Autodesk Inventor part; units mm, degrees
(part 3 of 3)
ref_plane "to_Bolt_1_6_YZ" through (-291.404, 0, -380) normal (1, 0, 0) x (0, 0, -1)
ref_plane "to_Bolt_1_6_ZX" through (-291.404, 0, -380) normal (0, 0, -1) x (0, 1, 0)
ref_plane "to_Bolt_1_60_XY" through (-198.5673, 0, -380) normal (0, 1, 0) x (1, 0, 0)
ref_plane "to_Bolt_1_60_YZ" through (-198.5673, 0, -380) normal (1, 0, 0) x (0, 0, -1)
ref_plane "to_Bolt_1_60_ZX" through (-198.5673, 0, -380) normal (0, 0, -1) x (0, 1, 0)
ref_plane "to_Bolt_1_61_XY" through (-196.8481, 0, -380) normal (0, 1, 0) x (1, 0, 0)
ref_plane "to_Bolt_1_61_YZ" through (-196.8481, 0, -380) normal (1, 0, 0) x (0, 0, -1)
ref_plane "to_Bolt_1_61_ZX" through (-196.8481, 0, -380) normal (0, 0, -1) x (0, 1, 0)
ref_plane "to_Bolt_1_62_XY" through (-195.1289, 0, -380) normal (0, 1, 0) x (1, 0, 0)
ref_plane "to_Bolt_1_62_YZ" through (-195.1289, 0, -380) normal (1, 0, 0) x (0, 0, -1)
ref_plane "to_Bolt_1_62_ZX" through (-195.1289, 0, -380) normal (0, 0, -1) x (0, 1, 0)
ref_plane "to_Bolt_1_63_XY" through (-193.4097, 0, -380) normal (0, 1, 0) x (1, 0, 0)
ref_plane "to_Bolt_1_63_YZ" through (-193.4097, 0, -380) normal (1, 0, 0) x (0, 0, -1)
ref_plane "to_Bolt_1_63_ZX" through (-193.4097, 0, -380) normal (0, 0, -1) x (0, 1, 0)
ref_plane "to_Bolt_1_64_XY" through (-191.6905, 0, -380) normal (0, 1, 0) x (1, 0, 0)
ref_plane "to_Bolt_1_64_YZ" through (-191.6905, 0, -380) normal (1, 0, 0) x (0, 0, -1)
ref_plane "to_Bolt_1_64_ZX" through (-191.6905, 0, -380) normal (0, 0, -1) x (0, 1, 0)
ref_plane "to_Bolt_1_65_XY" through (-189.9713, 0, -380) normal (0, 1, 0) x (1, 0, 0)
ref_plane "to_Bolt_1_65_YZ" through (-189.9713, 0, -380) normal (1, 0, 0) x (0, 0, -1)
ref_plane "to_Bolt_1_65_ZX" through (-189.9713, 0, -380) normal (0, 0, -1) x (0, 1, 0)
ref_plane "to_Bolt_1_66_XY" through (-188.2521, 0, -380) normal (0, 1, 0) x (1, 0, 0)
ref_plane "to_Bolt_1_66_YZ" through (-188.2521, 0, -380) normal (1, 0, 0) x (0, 0, -1)
ref_plane "to_Bolt_1_66_ZX" through (-188.2521, 0, -380) normal (0, 0, -1) x (0, 1, 0)
ref_plane "to_Bolt_1_67_XY" through (-186.533, 0, -380) normal (0, 1, 0) x (1, 0, 0)
ref_plane "to_Bolt_1_67_YZ" through (-186.533, 0, -380) normal (1, 0, 0) x (0, 0, -1)
ref_plane "to_Bolt_1_67_ZX" through (-186.533, 0, -380) normal (0, 0, -1) x (0, 1, 0)
ref_plane "to_Bolt_1_68_XY" through (-184.8138, 0, -380) normal (0, 1, 0) x (1, 0, 0)
ref_plane "to_Bolt_1_68_YZ" through (-184.8138, 0, -380) normal (1, 0, 0) x (0, 0, -1)
ref_plane "to_Bolt_1_68_ZX" through (-184.8138, 0, -380) normal (0, 0, -1) x (0, 1, 0)
ref_plane "to_Bolt_1_69_XY" through (-183.0946, 0, -380) normal (0, 1, 0) x (1, 0, 0)
ref_plane "to_Bolt_1_69_YZ" through (-183.0946, 0, -380) normal (1, 0, 0) x (0, 0, -1)
ref_plane "to_Bolt_1_69_ZX" through (-183.0946, 0, -380) normal (0, 0, -1) x (0, 1, 0)
ref_plane "to_Bolt_1_7_XY" through (-289.6848, 0, -380) normal (0, 1, 0) x (1, 0, 0)
ref_plane "to_Bolt_1_7_YZ" through (-289.6848, 0, -380) normal (1, 0, 0) x (0, 0, -1)
ref_plane "to_Bolt_1_7_ZX" through (-289.6848, 0, -380) normal (0, 0, -1) x (0, 1, 0)
ref_plane "to_Bolt_1_70_XY" through (-181.3754, 0, -380) normal (0, 1, 0) x (1, 0, 0)
ref_plane "to_Bolt_1_70_YZ" through (-181.3754, 0, -380) normal (1, 0, 0) x (0, 0, -1)
ref_plane "to_Bolt_1_70_ZX" through (-181.3754, 0, -380) normal (0, 0, -1) x (0, 1, 0)
ref_plane "to_Bolt_1_71_XY" through (-179.6562, 0, -380) normal (0, 1, 0) x (1, 0, 0)
ref_plane "to_Bolt_1_71_YZ" through (-179.6562, 0, -380) normal (1, 0, 0) x (0, 0, -1)
ref_plane "to_Bolt_1_71_ZX" through (-179.6562, 0, -380) normal (0, 0, -1) x (0, 1, 0)
ref_plane "to_Bolt_1_72_XY" through (-177.937, 0, -380) normal (0, 1, 0) x (1, 0, 0)
ref_plane "to_Bolt_1_72_YZ" through (-177.937, 0, -380) normal (1, 0, 0) x (0, 0, -1)
ref_plane "to_Bolt_1_72_ZX" through (-177.937, 0, -380) normal (0, 0, -1) x (0, 1, 0)
ref_plane "to_Bolt_1_73_XY" through (-176.2178, 0, -380) normal (0, 1, 0) x (1, 0, 0)
ref_plane "to_Bolt_1_73_YZ" through (-176.2178, 0, -380) normal (1, 0, 0) x (0, 0, -1)
ref_plane "to_Bolt_1_73_ZX" through (-176.2178, 0, -380) normal (0, 0, -1) x (0, 1, 0)
ref_plane "to_Bolt_1_74_XY" through (-174.4986, 0, -380) normal (0, 1, 0) x (1, 0, 0)
ref_plane "to_Bolt_1_74_YZ" through (-174.4986, 0, -380) normal (1, 0, 0) x (0, 0, -1)
ref_plane "to_Bolt_1_74_ZX" through (-174.4986, 0, -380) normal (0, 0, -1) x (0, 1, 0)
ref_plane "to_Bolt_1_75_XY" through (-172.7794, 0, -380) normal (0, 1, 0) x (1, 0, 0)
ref_plane "to_Bolt_1_75_YZ" through (-172.7794, 0, -380) normal (1, 0, 0) x (0, 0, -1)
ref_plane "to_Bolt_1_75_ZX" through (-172.7794, 0, -380) normal (0, 0, -1) x (0, 1, 0)
ref_plane "to_Bolt_1_76_XY" through (-171.0602, 0, -380) normal (0, 1, 0) x (1, 0, 0)
ref_plane "to_Bolt_1_76_YZ" through (-171.0602, 0, -380) normal (1, 0, 0) x (0, 0, -1)
ref_plane "to_Bolt_1_76_ZX" through (-171.0602, 0, -380) normal (0, 0, -1) x (0, 1, 0)
ref_plane "to_Bolt_1_77_XY" through (-169.341, 0, -380) normal (0, 1, 0) x (1, 0, 0)
ref_plane "to_Bolt_1_77_YZ" through (-169.341, 0, -380) normal (1, 0, 0) x (0, 0, -1)
ref_plane "to_Bolt_1_77_ZX" through (-169.341, 0, -380) normal (0, 0, -1) x (0, 1, 0)
ref_plane "to_Bolt_1_78_XY" through (-167.6218, 0, -380) normal (0, 1, 0) x (1, 0, 0)
ref_plane "to_Bolt_1_78_YZ" through (-167.6218, 0, -380) normal (1, 0, 0) x (0, 0, -1)
ref_plane "to_Bolt_1_78_ZX" through (-167.6218, 0, -380) normal (0, 0, -1) x (0, 1, 0)
ref_plane "to_Bolt_1_79_XY" through (-165.9026, 0, -380) normal (0, 1, 0) x (1, 0, 0)
ref_plane "to_Bolt_1_79_YZ" through (-165.9026, 0, -380) normal (1, 0, 0) x (0, 0, -1)
ref_plane "to_Bolt_1_79_ZX" through (-165.9026, 0, -380) normal (0, 0, -1) x (0, 1, 0)
ref_plane "to_Bolt_1_8_XY" through (-287.9656, 0, -380) normal (0, 1, 0) x (1, 0, 0)
ref_plane "to_Bolt_1_8_YZ" through (-287.9656, 0, -380) normal (1, 0, 0) x (0, 0, -1)
ref_plane "to_Bolt_1_8_ZX" through (-287.9656, 0, -380) normal (0, 0, -1) x (0, 1, 0)
ref_plane "to_Bolt_1_80_XY" through (-164.1834, 0, -380) normal (0, 1, 0) x (1, 0, 0)
ref_plane "to_Bolt_1_80_YZ" through (-164.1834, 0, -380) normal (1, 0, 0) x (0, 0, -1)
ref_plane "to_Bolt_1_80_ZX" through (-164.1834, 0, -380) normal (0, 0, -1) x (0, 1, 0)
ref_plane "to_Bolt_1_81_XY" through (-162.4642, 0, -380) normal (0, 1, 0) x (1, 0, 0)
ref_plane "to_Bolt_1_81_YZ" through (-162.4642, 0, -380) normal (1, 0, 0) x (0, 0, -1)
ref_plane "to_Bolt_1_81_ZX" through (-162.4642, 0, -380) normal (0, 0, -1) x (0, 1, 0)
ref_plane "to_Bolt_1_82_XY" through (-160.745, 0, -380) normal (0, 1, 0) x (1, 0, 0)
ref_plane "to_Bolt_1_82_YZ" through (-160.745, 0, -380) normal (1, 0, 0) x (0, 0, -1)
ref_plane "to_Bolt_1_82_ZX" through (-160.745, 0, -380) normal (0, 0, -1) x (0, 1, 0)
ref_plane "to_Bolt_1_83_XY" through (-159.0258, 0, -380) normal (0, 1, 0) x (1, 0, 0)
ref_plane "to_Bolt_1_83_YZ" through (-159.0258, 0, -380) normal (1, 0, 0) x (0, 0, -1)
ref_plane "to_Bolt_1_83_ZX" through (-159.0258, 0, -380) normal (0, 0, -1) x (0, 1, 0)
ref_plane "to_Bolt_1_84_XY" through (-157.3066, 0, -380) normal (0, 1, 0) x (1, 0, 0)
ref_plane "to_Bolt_1_84_YZ" through (-157.3066, 0, -380) normal (1, 0, 0) x (0, 0, -1)
ref_plane "to_Bolt_1_84_ZX" through (-157.3066, 0, -380) normal (0, 0, -1) x (0, 1, 0)
ref_plane "to_Bolt_1_85_XY" through (-155.5874, 0, -380) normal (0, 1, 0) x (1, 0, 0)
ref_plane "to_Bolt_1_85_YZ" through (-155.5874, 0, -380) normal (1, 0, 0) x (0, 0, -1)
ref_plane "to_Bolt_1_85_ZX" through (-155.5874, 0, -380) normal (0, 0, -1) x (0, 1, 0)
ref_plane "to_Bolt_1_86_XY" through (-153.8682, 0, -380) normal (0, 1, 0) x (1, 0, 0)
ref_plane "to_Bolt_1_86_YZ" through (-153.8682, 0, -380) normal (1, 0, 0) x (0, 0, -1)
ref_plane "to_Bolt_1_86_ZX" through (-153.8682, 0, -380) normal (0, 0, -1) x (0, 1, 0)
ref_plane "to_Bolt_1_87_XY" through (-152.149, 0, -380) normal (0, 1, 0) x (1, 0, 0)
ref_plane "to_Bolt_1_87_YZ" through (-152.149, 0, -380) normal (1, 0, 0) x (0, 0, -1)
ref_plane "to_Bolt_1_87_ZX" through (-152.149, 0, -380) normal (0, 0, -1) x (0, 1, 0)
ref_plane "to_Bolt_1_88_XY" through (-150.4298, 0, -380) normal (0, 1, 0) x (1, 0, 0)
ref_plane "to_Bolt_1_88_YZ" through (-150.4298, 0, -380) normal (1, 0, 0) x (0, 0, -1)
ref_plane "to_Bolt_1_88_ZX" through (-150.4298, 0, -380) normal (0, 0, -1) x (0, 1, 0)
ref_plane "to_Bolt_1_89_XY" through (-148.7106, 0, -380) normal (0, 1, 0) x (1, 0, 0)
ref_plane "to_Bolt_1_89_YZ" through (-148.7106, 0, -380) normal (1, 0, 0) x (0, 0, -1)
ref_plane "to_Bolt_1_89_ZX" through (-148.7106, 0, -380) normal (0, 0, -1) x (0, 1, 0)
ref_plane "to_Bolt_1_9_XY" through (-286.2464, 0, -380) normal (0, 1, 0) x (1, 0, 0)
ref_plane "to_Bolt_1_9_YZ" through (-286.2464, 0, -380) normal (1, 0, 0) x (0, 0, -1)
ref_plane "to_Bolt_1_9_ZX" through (-286.2464, 0, -380) normal (0, 0, -1) x (0, 1, 0)
ref_plane "to_Bolt_1_90_XY" through (-146.9914, 0, -380) normal (0, 1, 0) x (1, 0, 0)
ref_plane "to_Bolt_1_90_YZ" through (-146.9914, 0, -380) normal (1, 0, 0) x (0, 0, -1)
ref_plane "to_Bolt_1_90_ZX" through (-146.9914, 0, -380) normal (0, 0, -1) x (0, 1, 0)
ref_plane "to_Bolt_1_91_XY" through (-145.2722, 0, -380) normal (0, 1, 0) x (1, 0, 0)
ref_plane "to_Bolt_1_91_YZ" through (-145.2722, 0, -380) normal (1, 0, 0) x (0, 0, -1)
ref_plane "to_Bolt_1_91_ZX" through (-145.2722, 0, -380) normal (0, 0, -1) x (0, 1, 0)
ref_plane "to_Bolt_1_92_XY" through (-143.553, 0, -380) normal (0, 1, 0) x (1, 0, 0)
ref_plane "to_Bolt_1_92_YZ" through (-143.553, 0, -380) normal (1, 0, 0) x (0, 0, -1)
ref_plane "to_Bolt_1_92_ZX" through (-143.553, 0, -380) normal (0, 0, -1) x (0, 1, 0)
ref_plane "to_Bolt_1_93_XY" through (-141.8338, 0, -380) normal (0, 1, 0) x (1, 0, 0)
ref_plane "to_Bolt_1_93_YZ" through (-141.8338, 0, -380) normal (1, 0, 0) x (0, 0, -1)
ref_plane "to_Bolt_1_93_ZX" through (-141.8338, 0, -380) normal (0, 0, -1) x (0, 1, 0)
ref_plane "to_Bolt_1_94_XY" through (-140.1146, 0, -380) normal (0, 1, 0) x (1, 0, 0)
ref_plane "to_Bolt_1_94_YZ" through (-140.1146, 0, -380) normal (1, 0, 0) x (0, 0, -1)
ref_plane "to_Bolt_1_94_ZX" through (-140.1146, 0, -380) normal (0, 0, -1) x (0, 1, 0)
ref_plane "to_Bolt_1_95_XY" through (-138.3954, 0, -380) normal (0, 1, 0) x (1, 0, 0)
ref_plane "to_Bolt_1_95_YZ" through (-138.3954, 0, -380) normal (1, 0, 0) x (0, 0, -1)
ref_plane "to_Bolt_1_95_ZX" through (-138.3954, 0, -380) normal (0, 0, -1) x (0, 1, 0)
ref_plane "to_Bolt_1_96_XY" through (-136.6762, 0, -380) normal (0, 1, 0) x (1, 0, 0)
ref_plane "to_Bolt_1_96_YZ" through (-136.6762, 0, -380) normal (1, 0, 0) x (0, 0, -1)
ref_plane "to_Bolt_1_96_ZX" through (-136.6762, 0, -380) normal (0, 0, -1) x (0, 1, 0)
ref_plane "to_Bolt_1_97_XY" through (-134.957, 0, -380) normal (0, 1, 0) x (1, 0, 0)
ref_plane "to_Bolt_1_97_YZ" through (-134.957, 0, -380) normal (1, 0, 0) x (0, 0, -1)
ref_plane "to_Bolt_1_97_ZX" through (-134.957, 0, -380) normal (0, 0, -1) x (0, 1, 0)
ref_plane "to_Bolt_1_98_XY" through (-133.2378, 0, -380) normal (0, 1, 0) x (1, 0, 0)
ref_plane "to_Bolt_1_98_YZ" through (-133.2378, 0, -380) normal (1, 0, 0) x (0, 0, -1)
ref_plane "to_Bolt_1_98_ZX" through (-133.2378, 0, -380) normal (0, 0, -1) x (0, 1, 0)
ref_plane "to_Bolt_1_99_XY" through (-131.5186, 0, -380) normal (0, 1, 0) x (1, 0, 0)
ref_plane "to_Bolt_1_99_YZ" through (-131.5186, 0, -380) normal (1, 0, 0) x (0, 0, -1)
ref_plane "to_Bolt_1_99_ZX" through (-131.5186, 0, -380) normal (0, 0, -1) x (0, 1, 0)
ref_plane "to_Bolt_2_XY" through (300, 0, -380) normal (0, 1, 0) x (1, 0, 0)
ref_plane "to_Bolt_2_YZ" through (300, 0, -380) normal (1, 0, 0) x (0, 0, -1)
ref_plane "to_Bolt_2_ZX" through (300, 0, -380) normal (0, 0, -1) x (0, 1, 0)
ref_plane "to_Bolt_3_XY" through (-300, 0, 380) normal (0, 1, 0) x (1, 0, 0)
ref_plane "to_Bolt_3_YZ" through (-300, 0, 380) normal (1, 0, 0) x (0, 0, -1)
ref_plane "to_Bolt_3_ZX" through (-300, 0, 380) normal (0, 0, -1) x (0, 1, 0)
ref_plane "to_Bolt_4_XY" through (300, 0, 380) normal (0, 1, 0) x (1, 0, 0)
ref_plane "to_Bolt_4_YZ" through (300, 0, 380) normal (1, 0, 0) x (0, 0, -1)
ref_plane "to_Bolt_4_ZX" through (300, 0, 380) normal (0, 0, -1) x (0, 1, 0)
body "Solid1"
